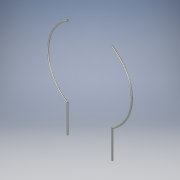
# Autodesk Inventor part: PossibleTopCapBallHolder
Saved by Autodesk Inventor 2017 (Build 210142000, 142)
## iProperties
Created: 2017-06-14
Part Number: PossibleTopCapBallHolder
Material: Silver
Document SubType Name: Modeling
Designer: User
Density: 10.49 g/cm^3
Appearance: Silver
Mass: 339.079 g
Surface Area: 205.387 cm^2
Volume: 32.324 cm^3
Author: User
Autodesk Inventor part; units mm, degrees
sketch "Sketch1" plane through (0, 0, 0) normal (0, 0, 1) x (1, 0, 0)
  arc A0 (-101.6, 161.1449) -> (-101.6, -161.1449) centre (0, 0) ccw
  arc A1 (101.6, -161.1449) -> (101.6, 161.1449) centre (0, 0) ccw
  point P0 (0, 0)
  constraints: 4 point on circle, 2 centre point
ref_plane "Work Plane5" through (101.6, 161.1449, 0) normal (-0.8459, 0.5333, 0) x (-0.5333, -0.8459, 0)
ref_plane "Work Plane6" through (-101.6, 161.1449, 0) normal (-0.8459, -0.5333, 0) x (0.5333, -0.8459, 0)
sketch "Sketch4" plane through (-101.6, 161.1449, 0) normal (-0.8459, -0.5333, 0) x (0.5333, -0.8459, 0)
  circle A0 centre (0, 0) radius 3.175
  point P0 (190.5, 0)
  dimension "d3" = 6.35
  constraints: 1 centre point
  measures "d3" diameter of A0
sketch "Sketch5" plane through (101.6, 161.1449, 0) normal (-0.8459, 0.5333, 0) x (-0.5333, -0.8459, 0)
  circle A0 centre (0, 0) radius 3.175
  point P0 (190.5, 0)
  dimension "d4" = 6.35
  constraints: 1 centre point
  measures "d4" diameter of A0
sweep "Sweep1" add profiles "Sketch4" path "Sketch1" path curves A0
sweep "Sweep2" add profiles "Sketch5" path "Sketch1" path curves A1
ref_plane "Work Plane7" through (0, 0, 0) normal (0, 0, -1) x (-1, 0, 0)
sketch "Sketch6" plane through (0, 0, 0) normal (0, 0, -1) x (-1, 0, 0)
  line L0 (99.9067, -158.4592) -> (103.2933, -163.8307) projected
  line L1 (101.6, -161.1449) -> (101.6, -288.1449)
  line L2 (-103.2933, -163.8307) -> (-99.9067, -158.4592) projected
  point P0 (0, 0)
  point P1 (-101.6, -161.1449)
  dimension "d9" = 127
  constraints: 2 end point, 2 midpoint, 1 vertical
  measures "d9" distance of L1.start L1.end
sketch "Sketch7" plane through (0, 0, 0) normal (0, 0, -1) x (-1, 0, 0)
  line L0 (-103.2933, -163.8307) -> (-99.9067, -158.4592) projected
  line L1 (-101.6, -161.1449) -> (-101.6, -288.1449)
  point P0 (0, 0)
  point P1 (-99.9067, -285.4592)
  dimension "d10" = 127
  dimension "d14" = 127
  constraints: 2 end point, 1 midpoint, 1 vertical
  measures "d10" distance of L0.end point (-99.907, -285.459)
  measures "d14" distance of L1.start L1.end
ref_plane "Work Plane8" through (-101.6, -288.1449, 0) normal (0, -1, 0) x (1, 0, 0)
sketch "Sketch8" plane through (-101.6, -288.1449, 0) normal (0, -1, 0) x (1, 0, 0)
  circle A0 centre (0, 0) radius 3.175
  point P0 (101.6, 0)
  dimension "d11" = 6.35
  constraints: 1 centre point
  measures "d11" diameter of A0
extrude "Extrusion1" add sketch "Sketch8" against normal blind 127
ref_plane "Work Plane10" through (101.6, -288.1449, 0) normal (0, -1, 0) x (1, 0, 0)
sketch "Sketch9" plane through (101.6, -288.1449, 0) normal (0, -1, 0) x (1, 0, 0)
  circle A0 centre (0, 0) radius 3.175
  point P0 (-101.6, 0)
  dimension "d15" = 6.35
  constraints: 1 centre point
  measures "d15" diameter of A0
extrude "Extrusion2" add sketch "Sketch9" against normal blind 127
body "Solid1"
